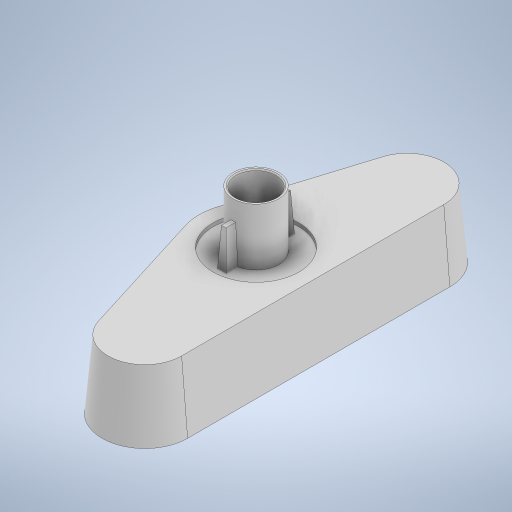
# Autodesk Inventor part: 4-3拔模
Saved by Autodesk Inventor 2024.2 (Build 282272000, 272)
## iProperties
Created: 2024-03-28
Part Number: 4-3拔模
Material: 一般
Document SubType Name: Modeling
Designer: User
Density: 1 g/cm^3
Appearance: 預設
Author: User
Autodesk Inventor part; units mm, degrees
ref_plane "YZ Plane" through (0, 0, 0) normal (1, 0, 0) x (0, 1, 0)
ref_plane "XZ Plane" through (0, 0, 0) normal (0, 1, 0) x (-1, 0, 0)
ref_plane "XY Plane" through (0, 0, 0) normal (0, 0, 1) x (1, 0, 0)
sketch "草圖1" plane through (0, 0, 0) normal (0, 1, 0) x (-1, 0, 0)
  arc A0 (10.5021, -3.2721) -> (10.5021, 3.2721) centre (0, 0) ccw
  line L0 (-11, 23) -> (-11, 0)
  line L1 (-11, 0) -> (-11, -23)
  arc A1 (-11, -23) -> (3.6605, -25.2309) centre (-3.5, -23) ccw
  line L2 (10.5021, -3.2721) -> (3.6605, -25.2309)
  arc A2 (3.6605, 25.2309) -> (-11, 23) centre (-3.5, 23) ccw
  line L3 (10.5021, 3.2721) -> (3.6605, 25.2309)
  dimension "d2" = 23
  dimension "d3" = 23
  constraints: 8 end point, 6 point on circle, 3 centre point, 1 coincident
  measures "d2" distance of L0.start L0.end
  measures "d3" distance of L0.end L1.end
extrude "擠出1" add sketch "草圖1" along normal blind 12
draft "面拔模1" angle 5 pull direction (0, 1, 0) faces at (11, 4, -7.6667) (11, 4, 15.3333) (-3.2211, 8, -26.3282) (10.9069, 8, 24.1782) (-5.941, 4, -17.9113) (-8.2216, 4, 10.5917) (-10.6979, 8, 2.5603) fixed edges at (11, 0, -11.5) (11, 0, 11.5) (4.6283, 0, -30.4146) (4.6283, 0, 30.4146) (-7.0813, 0, -14.2515) (-7.0813, 0, 14.2515) (-11, 0, 0)
sketch "草圖2" plane through (0, 12, 0) normal (0, 1, 0) x (1, 0, 0)
  circle A0 centre (0, 0) radius 7.5
  dimension "d8" = 15
  constraints: 1 centre point, 1 coincident
  measures "d8" diameter of A0
extrude "擠出2" cut sketch "草圖2" against normal blind 0.6
sketch "草圖3" plane through (0, 11.4, 0) normal (0, 1, 0) x (1, 0, 0)
  circle A0 centre (0, 0) radius 4
  dimension "d11" = 8
  constraints: 1 centre point, 1 coincident
  measures "d11" diameter of A0
extrude "擠出3" add sketch "草圖3" along normal blind 10
sketch "草圖4" plane through (0, 0, 0) normal (0, -1, 0) x (1, 0, 0)
  circle A0 centre (0, 0) radius 4 projected
  circle A1 centre (0, 0) radius 7.5 projected
  line L0 (0.75, 3.9291) -> (0.75, 6)
  line L1 (0.75, 6) -> (-0.75, 6)
  line L2 (-0.75, -6) -> (0.75, -6)
  line L3 (0.75, -6) -> (0.75, -3.9291)
  line L4 (-0.75, 6) -> (-0.75, 3.9291)
  line L5 (-0.75, -3.9291) -> (-0.75, -6)
  circle A2 centre (0, 0) radius 4
  dimension "d16" = 1.5
  dimension "d17" = 12
  dimension "d18" = 1.5
  constraints: 12 end point, 4 point on circle, 3 perpendicular, 1 centre point, 1 coincident, 1 concentric, 1 point on line, 1 vertical
  measures "d16" distance of L0.end L1.end
  measures "d17" distance of L1.end L2.start
  measures "d18" distance of L2.start L2.end
extrude "擠出4" add sketch "草圖4" against normal blind 18 separate body contours A0 L4 L1 L0 | L3 L2 L5 A0
draft "面拔模2" angle 3 pull direction (0, 1, 0) fixed plane through (6.2607, 11.4, -0.5983) normal (0, 1, 0) faces at (0.75, 6, -5.3097) (-0.25, 12, -6) (-0.75, 6, -4.6194)
draft "面拔模3" angle 3 pull direction (0, 1, 0) fixed plane through (6.2607, 11.4, -0.5983) normal (0, 1, 0) faces at (0.75, 6, 4.6194) (0.25, 12, 6) (-0.75, 12, 5.3097)
sketch "草圖5" plane through (0, 21.4, 0) normal (0, 1, 0) x (1, 0, 0)
  circle A0 centre (0, 0) radius 3.5
  dimension "d23" = 7
  constraints: 1 centre point, 1 coincident
  measures "d23" diameter of A0
extrude "擠出5" cut sketch "草圖5" against normal blind 15 bodies 1
chamfer "倒角1" distance 0.2 angle 45 1 edges at (-3.5, 21.4, 0)
